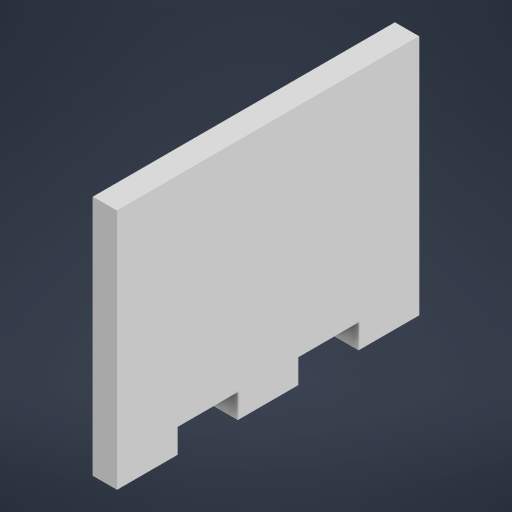
# Autodesk Inventor part: Langbektang houder
Saved by Autodesk Inventor 2023.2 (Build 272271000, 271)
## iProperties
Created: 2020-09-09
Part Number: Langbektang houder
Material: Generic
Document SubType Name: Modeling
Designer: nathan.bollaert
Density: 1 g/cm^3
Appearance: Default
Author: nathan.bollaert
Autodesk Inventor part; units mm, degrees
ref_plane "YZ Plane" through (0, 0, 0) normal (1, 0, 0) x (0, 1, 0)
ref_plane "XZ Plane" through (0, 0, 0) normal (0, 1, 0) x (-1, 0, 0)
ref_plane "XY Plane" through (0, 0, 0) normal (0, 0, 1) x (1, 0, 0)
sketch "Sketch1" plane through (0, 0, 0) normal (1, 0, 0) x (0, 1, 0)
  line L0 (0, 0) -> (-4, 0)
  line L1 (0, 0) -> (36, 0)
  line L2 (36, 0) -> (36, -50)
  line L3 (36, -50) -> (0, -50)
  line L4 (0, -50) -> (0, 0)
  line L5 (-4, 0) -> (-4, -10)
  line L6 (-4, -20) -> (-4, -30)
  line L7 (0, -20) -> (0, -10)
  line L8 (-4, -10) -> (0, -10)
  line L9 (0, -20) -> (-4, -20)
  line L10 (-4, -40) -> (-4, -50)
  line L11 (0, -40) -> (0, -30)
  line L12 (-4, -30) -> (0, -30)
  line L13 (0, -40) -> (-4, -40)
  line L14 (-4, -50) -> (0, -50)
  dimension "d230" = 36
  dimension "d231" = 50
  dimension "d236" = 10
  dimension "d240" = 10
  dimension "d241" = 4
  constraints: 30 end point, 12 equal length, 4 perpendicular, 3 vertical, 2 horizontal, 1 coincident
  measures "d230" distance of L2.end L3.end
  measures "d231" distance of L1.end L2.end
  measures "d236" distance of L5.end L6.start
  measures "d240" distance of L0.end L5.end
  measures "d241" distance between parallel lines of L4 L5
extrude "Extrusion1" add sketch "Sketch1" against normal blind 4
body "Solid5"
